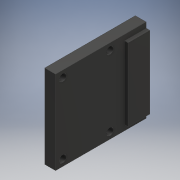
# Autodesk Inventor part: camera
Saved by Autodesk Inventor 2017 (Build 210142000, 142)
## iProperties
Part Number: camera
Material: Genérico
Document SubType Name: Modeling
Designer: Roberto
Density: 1 g/cm^3
Appearance: Valor por defecto
Author: Roberto
Autodesk Inventor part; units mm, degrees
ref_plane "YZ Plane" through (0, 0, 0) normal (1, 0, 0) x (0, 1, 0)
ref_plane "XZ Plane" through (0, 0, 0) normal (0, 1, 0) x (-1, 0, 0)
ref_plane "XY Plane" through (0, 0, 0) normal (0, 0, 1) x (1, 0, 0)
sketch "Boceto1" plane through (0, 0, 0) normal (1, 0, 0) x (0, 1, 0)
  line L0 (0, 0) -> (0, -2.3)
  line L1 (0, -2.3) -> (2.5, -2.3)
  line L2 (2.5, -2.3) -> (2.5, 0)
  line L3 (2.5, 0) -> (0, 0)
  line L4 (0, 0) -> (0.2, 0)
  line L5 (0.2, 0) -> (0.2, -0.18)
  circle A0 centre (0.2, -0.18) radius 0.1
  line L6 (0, 0) -> (1.5, 0)
  circle A1 centre (1.5, -0.18) radius 0.1
  circle A2 centre (0.2, -2.12) radius 0.1
  circle A3 centre (1.5, -2.12) radius 0.1
  line L7 (2.5, -0.15) -> (1.9, -0.15)
  line L8 (1.9, -0.15) -> (1.9, -2.15)
  line L9 (1.9, -2.15) -> (2.5, -2.15)
  dimension "d0" = 2.3
  dimension "d1" = 2.5
  dimension "d2" = 0.2
  dimension "d3" = 0.18
  dimension "d4" = 0.2
  dimension "d5" = 1.5
  dimension "d6" = 0.2
  dimension "d8" = 0.6
  constraints: 20 end point, 5 perpendicular, 4 centre point, 4 point on line, 1 coincident, 1 vertical
  measures "d0" distance of L0.start L0.end
  measures "d1" distance of L0.end L1.end
  measures "d2" distance of L0.start L4.end
  measures "d3" distance of L4.end L5.end
  measures "d4" diameter of A0
  measures "d5" distance of L0.start L6.end
  measures "d6" diameter of A1
  measures "d8" distance of L7.start L7.end
extrude "Extrusión1" add sketch "Boceto1" along normal blind 0.3
sketch "Boceto2" plane through (0.3, 0, 0) normal (1, 0, 0) x (0, 0, -1)
  line L0 (0, 0) -> (2.3, 0)
  line L1 (2.3, 0) -> (2.3, 2.5)
  line L2 (2.3, 2.5) -> (0, 2.5)
  line L3 (0, 2.5) -> (0, 0)
  line L4 (0, 0) -> (0, 0.2)
  line L5 (0, 0.2) -> (0.18, 0.2)
  circle A0 centre (0.18, 0.2) radius 0.1
  line L6 (0, 0) -> (0, 1.5)
  circle A1 centre (0.18, 1.5) radius 0.1
  circle A2 centre (2.12, 0.2) radius 0.1
  circle A3 centre (2.12, 1.5) radius 0.1
  line L7 (0.15, 2.5) -> (0.15, 1.9)
  line L8 (0.15, 1.9) -> (2.15, 1.9)
  line L9 (2.15, 1.9) -> (2.15, 2.5)
  line L10 (0, 0) -> (2.3, 0)
  line L11 (2.3, 0) -> (2.3, 2.5)
  line L12 (2.3, 2.5) -> (0, 2.5)
  line L13 (0, 2.5) -> (0, 0)
  line L14 (0, 0) -> (0, 0.2)
  line L15 (0, 0.2) -> (0.18, 0.2)
  circle A4 centre (0.18, 0.2) radius 0.1
  line L16 (0, 0) -> (0, 1.5)
  circle A5 centre (0.18, 1.5) radius 0.1
  circle A6 centre (2.12, 0.2) radius 0.1
  circle A7 centre (2.12, 1.5) radius 0.1
  line L17 (0.15, 2.5) -> (0.15, 1.9)
  line L18 (0.15, 1.9) -> (2.15, 1.9)
  line L19 (2.15, 1.9) -> (2.15, 2.5)
  dimension "d12" = 2.3
  dimension "d13" = 2.5
  dimension "d14" = 0.2
  dimension "d15" = 0.18
  dimension "d16" = 0.2
  dimension "d17" = 1.5
  dimension "d18" = 0.2
  dimension "d19" = 0.6
  dimension "d20" = 2.3
  dimension "d21" = 2.5
  dimension "d22" = 0.2
  dimension "d23" = 0.18
  dimension "d24" = 0.2
  dimension "d25" = 1.5
  dimension "d26" = 0.2
  dimension "d27" = 0.6
  constraints: 40 end point, 10 perpendicular, 8 centre point, 8 point on line, 2 coincident
  measures "d12" distance of L0.start L0.end
  measures "d13" distance of L0.end L2.start
  measures "d14" distance of L0.start L5.start
  measures "d15" distance of L5.start L5.end
  measures "d16" diameter of A0
  measures "d17" distance of L0.start L6.end
  measures "d18" diameter of A1
  measures "d19" distance of L7.start L8.start
  measures "d20" distance of L10.start L10.end
  measures "d21" distance of L10.end L12.start
  measures "d22" distance of L10.start L15.start
  measures "d23" distance of L15.start L15.end
  measures "d24" diameter of A4
  measures "d25" distance of L10.start L16.end
  measures "d26" diameter of A5
  measures "d27" distance of L17.start L18.start
extrude "Extrusión2" add sketch "Boceto2" along normal blind 0.1 contours L9 L8 L7 L2
sketch "Boceto3" plane through (0, 0, 0) normal (-1, 0, 0) x (0, 0, 1)
  line L0 (0, 0) -> (-2.3, 0) projected
  line L1 (-2.3, 0) -> (-1.5, 0)
  line L2 (-1.5, 0) -> (-1.5, 0.9)
  line L3 (-1.5, 0.9) -> (-0.75, 0.9)
  line L4 (-0.75, 0.9) -> (-0.75, 1.65)
  line L5 (-0.75, 1.65) -> (-1.5, 1.65)
  line L6 (-1.5, 1.65) -> (-1.5, 0.9)
  circle A0 centre (-1.125, 1.275) radius 0.275
  dimension "d30" = 0.8
  dimension "d31" = 0.9
  dimension "d32" = 0.75
  dimension "d33" = 0.75
  dimension "d34" = 0.75
  dimension "d35" = 0.55
  constraints: 12 end point, 3 perpendicular, 1 centre point, 1 point on line, 1 vertical
  measures "d30" distance of L0.end L1.end
  measures "d31" distance of L1.end L2.end
  measures "d32" distance of L2.end L3.end
  measures "d33" distance of L3.end L4.end
  measures "d34" distance of L4.end L5.end
  measures "d35" diameter of A0
extrude "Extrusión3" add sketch "Boceto3" along normal blind 0.2 contours L6 L5 L4 L3 | A0
sketch "Boceto4" plane through (-0.2, 0, 0) normal (-1, 0, 0) x (0, 0, 1)
  line L0 (-1.5, 0) -> (-1.5, 0.9)
  line L1 (-1.5, 0.9) -> (-0.75, 0.9)
  line L2 (-0.75, 0.9) -> (-0.75, 1.65)
  line L3 (-0.75, 1.65) -> (-1.5, 1.65)
  line L4 (-1.5, 1.65) -> (-1.5, 0.9)
  circle A0 centre (-1.125, 1.275) radius 0.275
  point P0 (0, 0)
  dimension "d38" = 0.9
  dimension "d39" = 0.75
  dimension "d40" = 0.75
  dimension "d41" = 0.75
  dimension "d42" = 0.55
  constraints: 10 end point, 2 perpendicular, 1 centre point, 1 vertical
  measures "d38" distance of L0.start L0.end
  measures "d39" distance of L0.end L1.end
  measures "d40" distance of L1.end L2.end
  measures "d41" distance of L2.end L3.end
  measures "d42" diameter of A0
extrude "Extrusión4" add sketch "Boceto4" along normal blind 0.2 contours A0
sketch "Boceto5" plane through (-0.4, 1.275, -1.125) normal (-1, 0, 0) x (0, 0, 1)
  circle A0 centre (0, 0) radius 0.275 projected
  circle A1 centre (0, 0) radius 0.15
  point P0 (1.125, -1.275)
  dimension "d45" = 0.125
  constraints: 1 centre point
  measures "d45" radial gap between concentric circles of A0 A1
extrude "Extrusión5" cut sketch "Boceto5" against normal blind 0.1 contours A1
